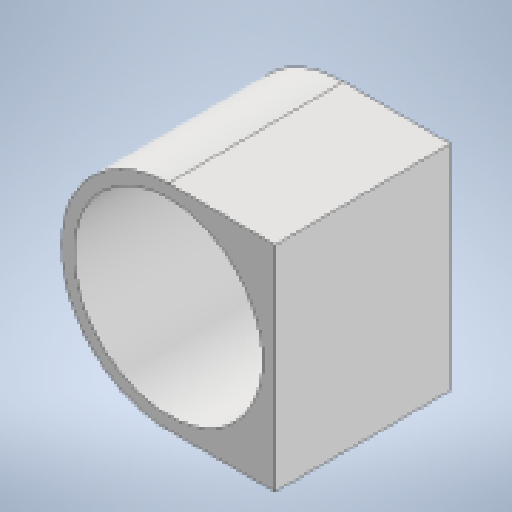
# Autodesk Inventor part: Arm_5
Saved by Autodesk Inventor 2023 (Build 270158000, 158)
## iProperties
Created: 2022-04-08
Part Number: Arm_5
Material: 一般
Document SubType Name: Modeling
Designer: device
Density: 1 g/cm^3
Appearance: 預設
Author: device
Autodesk Inventor part; units mm, degrees
ref_plane "YZ Plane" through (0, 0, 0) normal (1, 0, 0) x (0, 1, 0)
ref_plane "XZ Plane" through (0, 0, 0) normal (0, 1, 0) x (-1, 0, 0)
ref_plane "XY Plane" through (0, 0, 0) normal (0, 0, 1) x (1, 0, 0)
sketch "草圖1" plane through (0, 0, 0) normal (0, 0, 1) x (1, 0, 0)
  line L0 (0, 0) -> (-50, 0) construction
  line L1 (0, 25) -> (-50, 25)
  line L2 (-50, -25) -> (0, -25)
  arc A0 (0, -25) -> (0, 25) centre (0, 0) ccw
  arc A1 (-50, 25) -> (-50, -25) centre (-50, 0) ccw
  line L3 (-25, 25) -> (-25, -25)
  point P0 (-25, 0)
  point P1 (25, 0)
  point P2 (-75, 0)
  dimension "d0" = 50
  dimension "d1" = 100
  constraints: 10 end point, 6 point on circle, 4 tangent, 3 midpoint, 2 centre point, 1 horizontal, 1 parallel
  measures "d0" diameter of A1
  measures "d1" distance of point (25, 0) point (-75, 0)
extrude "擠出1" add sketch "草圖1" along normal mid plane 3 contours L3 L2 A1 L1
sketch "草圖2" plane through (0, 0, 1.5) normal (0, 0, 1) x (1, 0, 0)
  arc A0 (-50, 25) -> (-50, -25) centre (-50, 0) ccw projected
  circle A1 centre (-50, 0) radius 25
  circle A2 centre (-50, 0) radius 22
  line L0 (-50, -25) -> (-25, -25) projected
  line L1 (-25, -25) -> (-25, 25) projected
  line L2 (-25, 25) -> (-50, 25) projected
  arc A3 (-50, 25) -> (-50, -25) centre (-50, 0) ccw projected
  point P0 (0, 0)
  point P1 (-50, 25)
  point P2 (-50, -25)
  dimension "d4" = 3
  constraints: 1 centre point, 1 coincident, 1 vertical alignment, 2 other
extrude "擠出2" add sketch "草圖2" against normal blind 41
sketch "草圖3" plane through (-25, -25, -1.5) normal (1, 0, 0) x (0, 0, 1)
  line L0 (-38, -50) -> (3, -50) construction
  line L1 (-38, -50) -> (-38, 0) construction
  line L2 (-38, 0) -> (3, 0) construction
  circle A0 centre (-17.5, -25) radius 1.5
  circle A1 centre (-27.5, -25) radius 1.5
  circle A2 centre (-17.5, -35) radius 1.5
  circle A3 centre (-7.5, -25) radius 1.5
  circle A4 centre (-17.5, -15) radius 1.5
  line L3 (-17.5, -50) -> (-17.5, 0) construction
  line L4 (3, 0) -> (3, -50) projected
  point P0 (1.5, -25)
  point P1 (-17.5, -25)
  dimension "d7" = 3
  dimension "d10" = 360
  dimension "d12" = 10
  constraints: 5 centre point, 3 midpoint, 2 end point, 1 coincident, 1 equal radius, 9 other
  measures "d7" diameter of A0
  measures "d12" distance of A0.centre A1.centre
extrude "擠出3" cut sketch "草圖3" against normal up to surface
